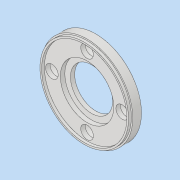
# Autodesk Inventor part: RadialBearingMountCover
Saved by Autodesk Inventor 2017 (Build 210142000, 142)
## iProperties
Created: 2016-11-28
Part Number: RadialBearingMountCover
Material: ABS Plastic
Document SubType Name: Modeling
Designer: techn
Density: 1.06 g/cm^3
Appearance: Smooth - White
Author: techn
Autodesk Inventor part; units mm, degrees
ref_plane "YZ Plane" through (0, 0, 0) normal (1, 0, 0) x (0, 1, 0)
ref_plane "XZ Plane" through (0, 0, 0) normal (0, 1, 0) x (-1, 0, 0)
ref_plane "XY Plane" through (0, 0, 0) normal (0, 0, 1) x (1, 0, 0)
sketch "Sketch1" plane through (0, 0, 0) normal (0, 0, 1) x (1, 0, 0)
  circle A0 centre (0, 0) radius 9.525
  line L0 (0, 0) -> (0, 15.875)
  circle A1 centre (0, 15.875) radius 1.5875
  circle A2 centre (-15.875, 0) radius 1.5875
  circle A3 centre (0, -15.875) radius 1.5875
  circle A4 centre (15.875, 0) radius 1.5875
  circle A5 centre (0, 0) radius 20.6375
  dimension "d0" = 19.05
  dimension "d1" = 15.875
  dimension "d2" = 3.175
  dimension "d5" = 360
  dimension "d7" = 41.275
  constraints: 6 centre point, 3 coincident, 2 end point, 1 vertical, 9 other
  measures "d0" diameter of A0
  measures "d1" distance of L0.start L0.end
  measures "d2" diameter of A1
  measures "d7" diameter of A5
extrude "Extrusion1" add sketch "Sketch1" against normal blind 1.905
chamfer "Chamfer1" distance 1.27 angle 45 4 edges at (-1.5875, 15.875, 0) (14.2875, 0, 0) (-1.5875, -15.875, 0) (-17.4625, 0, 0)
sketch "Sketch4" plane through (0, 0, 0) normal (0, 0, 1) x (1, 0, 0)
  circle A0 centre (0, -15.875) radius 2.8575 projected
  circle A1 centre (0, 15.875) radius 2.8575 projected
  circle A2 centre (0, 0) radius 9.525 projected
  circle A3 centre (0, 0) radius 20.6375 projected
  circle A4 centre (15.875, 0) radius 2.8575 projected
  circle A5 centre (-15.875, 0) radius 2.8575 projected
extrude "Extrusion3" add sketch "Sketch4" along normal blind 2.032
sketch "Sketch5" plane through (0, 0, 2.032) normal (0, 0, 1) x (1, 0, 0)
  circle A0 centre (0, 0) radius 12.065
  dimension "d17" = 24.13
  constraints: 1 centre point, 1 coincident
  measures "d17" diameter of A0
extrude "Extrusion4" cut sketch "Sketch5" against normal blind 2.032
sketch "Sketch6" plane through (0, 0, 2.032) normal (0, 0, 1) x (1, 0, 0)
  circle A0 centre (0, 0) radius 19.2405
  circle A1 centre (0, 0) radius 20.0025
  dimension "d20" = 38.481
  dimension "d21" = 40.005
  constraints: 2 centre point, 2 coincident
  measures "d20" diameter of A0
  measures "d21" diameter of A1
extrude "Extrusion5" add sketch "Sketch6" along normal blind 1.27
body "Solid1"
